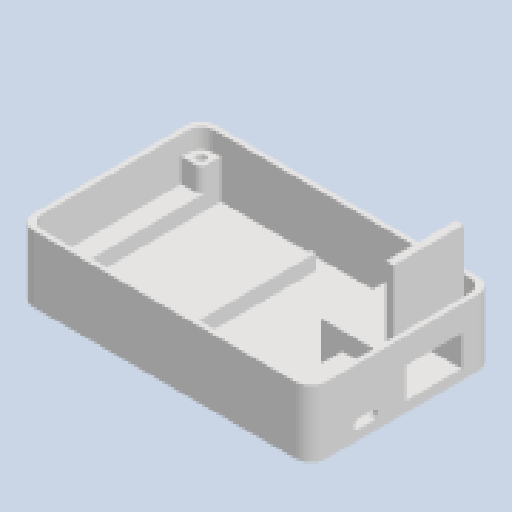
# Autodesk Inventor part: bottom
Saved by Autodesk Inventor 2025.2 (Build 292293000, 293)
## iProperties
Created: 2024-03-13
Part Number: bottom
Material: Generic
Document SubType Name: Modeling
Designer: mirun
Density: 1 g/cm^3
Appearance: Default
Author: mirun
Autodesk Inventor part; units mm, degrees
ref_plane "YZ Plane" through (0, 0, 0) normal (1, 0, 0) x (0, 1, 0)
ref_plane "XZ Plane" through (0, 0, 0) normal (0, 1, 0) x (-1, 0, 0)
sketch "Sketch1" plane through (0, 0, 0) normal (0, 1, 0) x (-1, 0, 0)
  line L0 (-55.26, 33.75) -> (55.26, 33.75)
  line L1 (55.26, 33.75) -> (55.26, -33.75)
  line L2 (55.26, -33.75) -> (-55.26, -33.75)
  line L3 (-55.26, -33.75) -> (-55.26, 33.75)
  line L4 (-55.26, 33.75) -> (55.26, -33.75) construction
  line L5 (55.26, 33.75) -> (-55.26, -33.75) construction
  point P0 (0, 0)
  dimension "d0" = 110.52
  dimension "d1" = 67.5
  constraints: 12 end point, 2 midpoint, 2 parallel, 1 horizontal, 1 perpendicular
  measures "d0" distance of L1.end L2.end
  measures "d1" distance between parallel lines of L2 L0
extrude "Extrusion1" add sketch "Sketch1" along normal blind 3
fillet "Fillet1" radius 5.25 4 edges at (-55.26, 1.5, 33.75) (55.26, 1.5, 33.75) (55.26, 1.5, -33.75) (-55.26, 1.5, -33.75)
sketch "Sketch2" plane through (0, 0, 0) normal (0, -1, 0) x (1, 0, 0)
  arc A0 (-55.26, -28.5) -> (-50.01, -33.75) centre (-50.01, -28.5) ccw construction
  line L0 (50.01, -33.75) -> (-50.01, -33.75) construction
  arc A1 (50.01, -33.75) -> (55.26, -28.5) centre (50.01, -28.5) ccw construction
  line L1 (55.26, 28.5) -> (55.26, -28.5) construction
  arc A2 (55.26, 28.5) -> (50.01, 33.75) centre (50.01, 28.5) ccw construction
  line L2 (-50.01, 33.75) -> (50.01, 33.75) construction
  arc A3 (-50.01, 33.75) -> (-55.26, 28.5) centre (-50.01, 28.5) ccw construction
  line L3 (-55.26, -28.5) -> (-55.26, 28.5) construction
  circle A4 centre (-50.01, 28.5) radius 5.25
  line L4 (-50.01, 33.75) -> (50.01, 33.75) construction
  line L5 (-50.01, 33.75) -> (50.01, 33.75)
  line L6 (-55.26, 28.5) -> (-55.26, -28.5)
  circle A5 centre (-50.01, -28.5) radius 5.25
  line L7 (-50.01, -33.75) -> (50.01, -33.75)
  circle A6 centre (50.01, -28.5) radius 5.25
  line L8 (55.26, 28.5) -> (55.26, -28.5)
  circle A7 centre (50.01, 28.5) radius 5.25
  line L9 (51.01, 35.75) -> (-51.01, 35.75)
  line L10 (-57.26, 29.5) -> (-57.26, -29.5)
  line L11 (-51.01, -35.75) -> (51.01, -35.75)
  line L12 (57.26, -29.5) -> (57.26, 29.5)
  line L13 (57.26, 35.75) -> (-57.26, -35.75) construction
  line L14 (-57.26, 35.75) -> (57.26, -35.75) construction
  arc A8 (-51.01, 35.75) -> (-57.26, 29.5) centre (-51.01, 29.5) ccw
  arc A9 (-57.26, -29.5) -> (-51.01, -35.75) centre (-51.01, -29.5) ccw
  arc A10 (51.01, -35.75) -> (57.26, -29.5) centre (51.01, -29.5) ccw
  arc A11 (57.26, 29.5) -> (51.01, 35.75) centre (51.01, 29.5) ccw
  point P0 (0, 0)
  point P1 (55.26, -28.5)
  point P2 (50.01, 33.75)
  dimension "d5" = 2
  dimension "d6" = 2
  dimension "d7" = 6.25
  dimension "d8" = 6.25
  constraints: 20 end point, 11 tangent, 9 point on circle, 8 point on line, 5 centre point, 5 equal length, 4 coincident, 3 equal radius, 2 midpoint, 2 vertical, 1 horizontal, 1 perpendicular, 9 other
  measures "d5" distance between parallel lines of L10 L3
  measures "d6" distance between parallel lines of L2 L9
  measures "d7" radius of A8
  measures "d8" radius of A9
extrude "Extrusion2" add sketch "Sketch2" against normal blind 26
sketch "Sketch3" plane through (55.26, 3, 28.5) normal (-1, 0, 0) x (0, 0, 1)
  line L0 (0, 0) -> (-57, 0) construction
  line L1 (-57, 23) -> (0, 23) construction
  line L2 (-54.5, 0) -> (-27, 0)
  line L3 (-27, 0) -> (-27, 47.408)
  line L4 (-27, 47.408) -> (-54.5, 47.408)
  line L5 (-54.5, 47.408) -> (-54.5, 0)
  line L6 (-62.25, 0) -> (-62.25, 23) construction
  point P0 (-28.5, -3)
  point P1 (-54.5, 23.704)
  point P2 (-40.75, 47.408)
  dimension "d11" = 7.75
  dimension "d12" = 27.5
  dimension "d13" = 24.408
  constraints: 8 end point, 2 midpoint, 2 parallel, 1 horizontal, 1 perpendicular, 1 point on line
  measures "d11" distance from line of point (-54.5, 23.704) L6
  measures "d12" distance between parallel lines of L3 L5
  measures "d13" distance from line of point (-40.75, 47.408) L1
extrude "Extrusion3" add sketch "Sketch3" along normal blind 3
sketch "Sketch4" plane through (0, 3, 0) normal (0, 1, 0) x (1, 0, 0)
  arc A0 (55.26, 28.5) -> (50.01, 33.75) centre (50.01, 28.5) ccw construction
  line L0 (50.01, 33.75) -> (-50.01, 33.75) construction
  line L1 (-50.01, -33.75) -> (50.01, -33.75) construction
  arc A1 (50.01, -33.75) -> (55.26, -28.5) centre (50.01, -28.5) ccw construction
  line L2 (55.26, -28.5) -> (55.26, -1.5) construction
  circle A2 centre (50.01, 28.5) radius 2.5
  circle A3 centre (50.01, -28.5) radius 2.5
  line L3 (47.51, -28.5) -> (47.51, -33.75)
  line L4 (55.26, -26) -> (50.01, -26)
  line L5 (0, 0) -> (0, -21.4582)
  line L6 (0, 0) -> (16.5599, 0)
  line L7 (47.51, 28.5) -> (47.51, 33.75)
  line L8 (55.26, 26) -> (50.01, 26)
  circle A4 centre (-50.01, 28.5) radius 2.5
  circle A5 centre (-50.01, -28.5) radius 2.5
  line L9 (-47.51, -28.5) -> (-47.51, -33.75)
  line L10 (-55.26, -26) -> (-50.01, -26)
  line L11 (-47.51, 28.5) -> (-47.51, 33.75)
  line L12 (-55.26, 26) -> (-50.01, 26)
  line L13 (55.26, 28.5) -> (55.26, -28.5)
  line L14 (50.01, 33.75) -> (5.9104, 33.75)
  arc A6 (55.26, 28.5) -> (50.01, 33.75) centre (50.01, 28.5) ccw
  arc A7 (50.01, -33.75) -> (55.26, -28.5) centre (50.01, -28.5) ccw
  line L15 (50.01, -33.75) -> (5.9104, -33.75)
  line L16 (-55.26, 26) -> (-55.26, 28.5) construction
  arc A8 (-50.01, 33.75) -> (-55.26, 28.5) centre (-50.01, 28.5) ccw construction
  line L17 (-50.01, 33.75) -> (50.01, 33.75) construction
  arc A9 (-55.26, -28.5) -> (-50.01, -33.75) centre (-50.01, -28.5) ccw construction
  line L18 (-55.26, -28.5) -> (-55.26, -1.5) construction
  line L19 (-55.26, 28.5) -> (-55.26, -28.5)
  line L20 (-50.01, 33.75) -> (-5.9104, 33.75)
  arc A10 (-50.01, 33.75) -> (-55.26, 28.5) centre (-50.01, 28.5) ccw
  arc A11 (-55.26, -28.5) -> (-50.01, -33.75) centre (-50.01, -28.5) ccw
  line L21 (-50.01, -33.75) -> (-5.9104, -33.75)
  point P0 (-47.51, 28.5)
  dimension "d16" = 5
  dimension "d17" = 5
  constraints: 38 end point, 30 symmetric about line, 18 point on circle, 10 centre point, 9 point on line, 4 coincident, 3 tangent, 2 horizontal, 1 collinear, 1 perpendicular, 1 vertical, 6 other
  measures "d16" diameter of A3
  measures "d17" diameter of A2
extrude "Extrusion4" add sketch "Sketch4" along normal blind 15.25
ref_plane "Work Plane1" through (0, 11.25, 0) normal (0, 1, 0) x (1, 0, 0)
sketch "Sketch5" plane through (0, 3, 0) normal (0, 1, 0) x (1, 0, 0)
  line L0 (-47.51, -33.75) -> (47.51, -33.75) construction
  arc A0 (-55.26, -28.5) -> (-50.01, -33.75) centre (-50.01, -28.5) ccw construction
  line L1 (-47.51, 28.5) -> (-55.26, 28.5)
  line L2 (-55.26, 28.5) -> (-55.26, -28.5)
  line L3 (-55.26, -28.5) -> (-47.51, -28.5)
  line L4 (-47.51, -28.5) -> (-47.51, 28.5)
  line L5 (-7.51, -33.75) -> (-5.51, -33.75)
  line L6 (-5.51, -33.75) -> (-5.51, 28.75)
  line L7 (-5.51, 28.75) -> (-7.51, 28.75)
  line L8 (-7.51, 28.75) -> (-7.51, -33.75)
  line L9 (-1.51, -33.75) -> (0.49, -33.75)
  dimension "d21" = 2
  dimension "d22" = 40
  constraints: 18 end point, 4 parallel, 3 horizontal, 2 perpendicular, 2 point on line
  measures "d21" distance of L7.end L6.end
  measures "d22" distance between parallel lines of L8 L4
extrude "Extrusion5" add sketch "Sketch5" along normal blind 6
sketch "Sketch6" plane through (0, 3, 0) normal (0, 1, 0) x (1, 0, 0)
  line L0 (55.26, -1.5) -> (52.26, -1.5) construction
  line L1 (52.26, 26) -> (27.26, 26)
  line L2 (27.26, 26) -> (27.26, -1.5)
  line L3 (27.26, -1.5) -> (52.26, -1.5)
  line L4 (52.26, -1.5) -> (52.26, 26)
  line L5 (57.26, -29.5) -> (57.26, 29.5) construction
  point P0 (0, 0)
  point P1 (27.26, 12.25)
  dimension "d29" = 30
  constraints: 8 end point, 2 parallel, 1 horizontal, 1 midpoint, 1 perpendicular, 1 point on line
  measures "d29" distance from line of L5 point (27.26, 12.25)
extrude "Extrusion6" add sketch "Sketch6" along normal up to surface (15.25 mm away)
sketch "Sketch7" plane through (57.26, 0, 29.5) normal (1, 0, 0) x (0, 0, -1)
  line L0 (59, 0) -> (0, 0) construction
  line L1 (0, 26) -> (59, 26) construction
  line L2 (48.75, 5.5) -> (34.75, 5.5)
  line L3 (34.75, 5.5) -> (34.75, 14.5)
  line L4 (34.75, 14.5) -> (48.75, 14.5)
  line L5 (48.75, 14.5) -> (48.75, 5.5)
  line L6 (48.75, 5.5) -> (34.75, 14.5) construction
  line L7 (34.75, 5.5) -> (48.75, 14.5) construction
  circle A0 centre (41.75, 10) radius 3.5
  line L8 (30.75, 16) -> (52.75, 16)
  line L9 (52.75, 16) -> (52.75, 4)
  line L10 (52.75, 4) -> (30.75, 4)
  line L11 (30.75, 4) -> (30.75, 16)
  line L12 (30.75, 16) -> (52.75, 4) construction
  line L13 (52.75, 16) -> (30.75, 4) construction
  line L14 (52.75, 16) -> (52.75, 26)
  line L15 (55.5, 50.408) -> (55.5, 18.25) construction
  line L16 (55.5, 26) -> (52.75, 26)
  line L17 (28, 26) -> (28, 50.408) construction
  line L18 (28, 26) -> (30.75, 26)
  line L19 (30.75, 16) -> (30.75, 26)
  point P0 (29.5, 0)
  dimension "d32" = 14
  dimension "d33" = 9
  dimension "d34" = 7
  dimension "d35" = 22
  dimension "d36" = 12
  dimension "d37" = 4
  constraints: 32 end point, 4 midpoint, 4 parallel, 4 point on line, 3 perpendicular, 2 collinear, 2 horizontal, 1 centre point, 1 coincident, 1 vertical
  measures "d32" distance of L3.end L4.end
  measures "d33" distance of L2.end L3.end
  measures "d34" diameter of A0
  measures "d35" distance of L9.end L10.end
  measures "d36" distance of L8.end L9.end
  measures "d37" distance between parallel lines of L10 L0
extrude "Extrusion7" cut sketch "Sketch7" against normal blind 13 contours L2 L3 L4 L5 | A0 | L8 L9 L10 L11
extrude "Extrusion8" cut sketch "Sketch7" against normal blind 20 contours A0
extrude "Extrusion9" cut sketch "Sketch7" against normal up to surface (10 mm away) from surface at -20 contours L2 L3 L4 L5 | A0
sketch "Sketch8" plane through (0, 3, 0) normal (0, 1, 0) x (1, 0, 0)
  line L0 (55.26, -1.5) -> (27.26, -1.5) construction
  line L1 (47.51, 33.75) -> (-47.51, 33.75) construction
  line L2 (-5.51, 28.75) -> (-5.51, -33.75) construction
  line L3 (-1.51, 25.75) -> (16.49, 25.75)
  line L4 (16.49, 25.75) -> (16.49, -1.75)
  line L5 (16.49, -1.75) -> (-1.51, -1.75)
  line L6 (-1.51, -1.75) -> (-1.51, 25.75)
  line L7 (-3.51, -8.5) -> (31.49, -8.5)
  line L8 (31.49, -8.5) -> (31.49, -27)
  line L9 (31.49, -27) -> (-3.51, -27)
  line L10 (-3.51, -27) -> (-3.51, -8.5)
  line L11 (57.26, -29.5) -> (57.26, 29.5) construction
  line L12 (-4.51, -22.25) -> (3.49, -22.25)
  line L13 (3.49, -22.25) -> (3.49, -13.25)
  line L14 (3.49, -13.25) -> (-4.51, -13.25)
  line L15 (-4.51, -13.25) -> (-4.51, -22.25)
  line L16 (-4.51, -22.25) -> (3.49, -13.25) construction
  line L17 (3.49, -22.25) -> (-4.51, -13.25) construction
  line L18 (25.49, -23.25) -> (31.49, -23.25)
  line L19 (31.49, -23.25) -> (31.49, -12.25)
  line L20 (31.49, -12.25) -> (25.49, -12.25)
  line L21 (25.49, -12.25) -> (25.49, -23.25)
  line L22 (25.49, -23.25) -> (31.49, -12.25) construction
  line L23 (31.49, -23.25) -> (25.49, -12.25) construction
  circle A0 centre (27.49, -22.25) radius 0.75
  point P0 (0, 0)
  point P1 (-0.51, -17.75)
  point P2 (-4.51, -17.75)
  point P3 (-3.51, -17.75)
  point P4 (28.49, -17.75)
  point P5 (31.49, -17.75)
  dimension "d44" = 18
  dimension "d45" = 27.5
  dimension "d46" = 8
  dimension "d48" = 35
  dimension "d49" = 18.5
  dimension "d52" = 7
  dimension "d59" = 2
  dimension "d60" = 4
  dimension "d75" = 1
  dimension "d76" = 9
  dimension "d77" = 8
  dimension "d78" = 11
  dimension "d79" = 6
  dimension "d80" = 1.5
  dimension "d81" = 1
  dimension "d82" = 2
  constraints: 40 end point, 8 parallel, 7 midpoint, 4 horizontal, 4 perpendicular, 2 horizontal alignment, 1 centre point, 1 point on line
  measures "d44" distance of L4.end L5.end
  measures "d45" distance of L3.end L4.end
  measures "d46" distance between parallel lines of L1 L3
  measures "d48" distance of L8.end L9.end
  measures "d49" distance between parallel lines of L9 L7
  measures "d52" distance between parallel lines of L7 L0
  measures "d59" distance between parallel lines of L10 L2
  measures "d60" distance between parallel lines of L2 L6
  measures "d75" distance of point (-4.51, -17.75) point (-3.51, -17.75)
  measures "d76" distance between parallel lines of L12 L14
  measures "d77" distance between parallel lines of L15 L13
  measures "d78" distance between parallel lines of L18 L20
  measures "d79" distance between parallel lines of L21 L8
  measures "d80" diameter of A0
  measures "d81" distance from line of L18 A0.centre
  measures "d82" distance from line of L21 A0.centre
sketch "Sketch9" plane through (55.26, 26, 1.5) normal (0, 0, 1) x (1, 0, 0)
  line L0 (-3, -7.75) -> (-28, -7.75) construction
  line L1 (0, -23) -> (-28, -23) construction
  line L2 (-20, -14.75) -> (-10, -14.75)
  line L3 (-10, -14.75) -> (-10, -17.5)
  line L4 (-10, -17.5) -> (-20, -17.5)
  line L5 (-20, -17.5) -> (-20, -14.75)
  line L6 (2, -22) -> (2, -10) construction
  point P0 (-55.26, -26)
  point P1 (-20, -16.125)
  point P2 (-10, -16.125)
  point P3 (2, -16)
  point P4 (-15, -14.75)
  dimension "d53" = 7
  dimension "d54" = 5.5
  dimension "d55" = 10
  dimension "d56" = 17
  constraints: 8 end point, 4 midpoint, 2 parallel, 1 horizontal, 1 perpendicular
  measures "d53" distance between parallel lines of L2 L0
  measures "d54" distance between parallel lines of L1 L4
  measures "d55" distance of point (-20, -16.125) point (-10, -16.125)
  measures "d56" horizontal distance of point (2, -16) point (-15, -14.75)
extrude "Extrusion10" add sketch "Sketch9" along normal up to surface (32.25 mm away)
sketch "Sketch10" plane through (57.26, 0, 29.5) normal (1, 0, 0) x (0, 0, -1)
  line L0 (12.25, 5.5) -> (18.25, 5.5) construction
  line L1 (12.25, 3.75) -> (18.25, 3.75)
  line L2 (18.25, 7.25) -> (12.25, 7.25)
  arc A0 (12.25, 7.25) -> (12.25, 3.75) centre (12.25, 5.5) ccw
  arc A1 (18.25, 3.75) -> (18.25, 7.25) centre (18.25, 5.5) ccw
  line L3 (3.5, 3) -> (3.5, 18.25) construction
  line L4 (3.5, 3) -> (28, 3) construction
  point P0 (29.5, 0)
  point P1 (15.25, 5.5)
  point P2 (20, 5.5)
  point P3 (10.5, 5.5)
  dimension "d61" = 3.5
  dimension "d62" = 9.5
  dimension "d63" = 7
  dimension "d64" = 0.75
  constraints: 8 end point, 6 point on circle, 4 tangent, 2 centre point, 1 horizontal, 1 midpoint, 1 parallel
  measures "d61" diameter of A1
  measures "d62" distance of point (20, 5.5) point (10.5, 5.5)
  measures "d63" distance from line of point (10.5, 5.5) L3
  measures "d64" distance between parallel lines of L1 L4
extrude "Extrusion11" cut sketch "Sketch10" against normal blind 10
sketch "Sketch11" plane through (0, 3, 0) normal (0, 1, 0) x (1, 0, 0)
  line L0 (55.26, -26) -> (55.26, -1.5) construction
  line L1 (48.76, -8) -> (55.26, -8)
  line L2 (55.26, -8) -> (55.26, -20.5)
  line L3 (55.26, -20.5) -> (48.76, -20.5)
  line L4 (48.76, -20.5) -> (48.76, -8)
  line L5 (48.76, -8) -> (55.26, -20.5) construction
  line L6 (55.26, -8) -> (48.76, -20.5) construction
  line L7 (45.26, -1.5) -> (45.26, -33.75) construction
  line L8 (48.76, -8) -> (45.26, -8)
  line L9 (45.26, -8) -> (45.26, -6)
  line L10 (45.26, -6) -> (48.76, -6)
  line L11 (48.76, -6) -> (48.76, -8)
  line L12 (48.76, -20.5) -> (45.26, -20.5)
  line L13 (45.26, -20.5) -> (45.26, -22.5)
  line L14 (45.26, -22.5) -> (48.76, -22.5)
  line L15 (48.76, -22.5) -> (48.76, -20.5)
  line L16 (50.01, -26) -> (55.26, -26) projected
  point P0 (0, 0)
  point P1 (52.01, -14.25)
  point P2 (55.26, -13.75)
  point P3 (55.26, -14.25)
  dimension "d67" = 12.5
  dimension "d68" = 6.5
  dimension "d69" = 2
  dimension "d70" = 2
  dimension "d102" = 11.75
  constraints: 28 end point, 6 parallel, 4 midpoint, 3 horizontal, 3 point on line, 2 perpendicular
  measures "d67" distance between parallel lines of L3 L1
  measures "d68" distance between parallel lines of L0 L4
  measures "d69" distance of L8.end L9.end
  measures "d70" distance of L13.end L12.end
  measures "d102" distance from line of L16 point (55.26, -14.25)
extrude "Extrusion12" cut sketch "Sketch11" against normal blind 2 contours L15 L14 L13 L12 | L8 L9 L10 L11
sketch "Sketch12" plane through (0, 3, 0) normal (0, 1, 0) x (1, 0, 0)
  line L0 (35.26, -1.5) -> (35.26, -33.75) construction
  line L1 (35.26, -1.5) -> (45.26, -1.5)
  line L2 (45.26, -1.5) -> (45.26, -8)
  line L3 (45.26, -8) -> (35.26, -8)
  line L4 (35.26, -8) -> (35.26, -1.5)
  line L5 (35.26, -33.75) -> (45.26, -33.75)
  line L6 (45.26, -33.75) -> (45.26, -20.5)
  line L7 (45.26, -20.5) -> (35.26, -20.5)
  line L8 (35.26, -20.5) -> (35.26, -33.75)
  point P0 (0, 0)
  constraints: 16 end point, 4 parallel, 2 horizontal, 2 perpendicular
extrude "Extrusion13" add sketch "Sketch12" along normal up to surface (8.25 mm away)
extrude "Extrusion14" cut sketch "Sketch8" against normal blind 1.5 contours L14 L13 L12 L10 | L10 L12 L15 L14 | L8 L18 L21 L20 | A0
extrude "Extrusion15" cut sketch "Sketch8" against normal through all contours A0
sketch "Sketch14" plane through (0, 0, 0) normal (0, -1, 0) x (1, 0, 0)
  arc A0 (51.01, -35.75) -> (57.26, -29.5) centre (51.01, -29.5) ccw projected
  arc A1 (55.26, 28.5) -> (50.01, 33.75) centre (50.01, 28.5) ccw projected
  arc A2 (57.26, 29.5) -> (51.01, 35.75) centre (51.01, 29.5) ccw projected
  arc A3 (-51.01, 35.75) -> (-57.26, 29.5) centre (-51.01, 29.5) ccw projected
  arc A4 (-50.01, 33.75) -> (-55.26, 28.5) centre (-50.01, 28.5) ccw projected
  arc A5 (-57.26, -29.5) -> (-51.01, -35.75) centre (-51.01, -29.5) ccw projected
  arc A6 (-55.26, -28.5) -> (-50.01, -33.75) centre (-50.01, -28.5) ccw projected
  arc A7 (50.01, -33.75) -> (55.26, -28.5) centre (50.01, -28.5) ccw projected
  point P0 (0, 0)
  constraints: 8 coincident
hole "Hole2" at (51.01, 0, -29.5) at (-51.01, 0, -29.5) at (-51.01, 0, 29.5) at (51.01, 0, 29.5) direction (0, 1, 0) diameter 3.4 end through all counterbore diameter 7 counterbore depth 4
body "Solid1"
